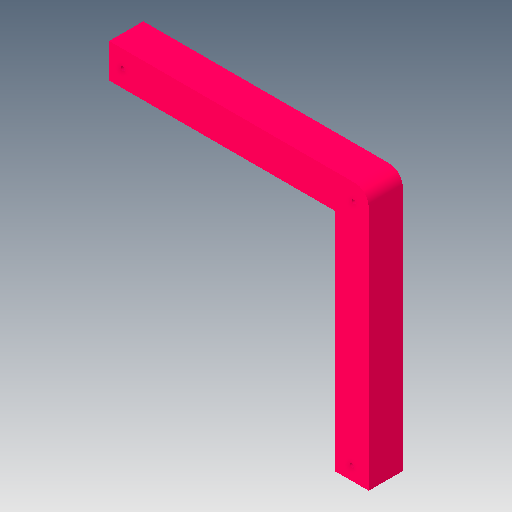
# Autodesk Inventor part: l almini
Saved by Autodesk Inventor 2018 (Build 220112000, 112)
## iProperties
Created: 2019-12-19
Part Number: l almini
Material: Generic
Document SubType Name: Modeling
Designer: Ibnu
Density: 1 g/cm^3
Appearance: Default
Mass: 220.808 g
Surface Area: 372.642 cm^2
Volume: 220.808 cm^3
Author: Ibnu
Autodesk Inventor part; units mm, degrees
ref_plane "YZ Plane" through (0, 0, 0) normal (1, 0, 0) x (0, 1, 0)
ref_plane "XZ Plane" through (0, 0, 0) normal (0, 1, 0) x (-1, 0, 0)
ref_plane "XY Plane" through (0, 0, 0) normal (0, 0, 1) x (1, 0, 0)
sketch "Sketch1" plane through (0, 0, 0) normal (0, 0, 1) x (1, 0, 0)
  line L0 (0, 0) -> (0, 25)
  line L1 (0, 25) -> (165, 25)
  line L2 (165, 0) -> (0, 0)
  line L3 (190, 0) -> (190, -165)
  line L4 (190, -165) -> (165, -165)
  line L5 (165, -165) -> (165, 0)
  line L6 (165, 25) -> (180, 25)
  line L7 (190, 15) -> (190, 0)
  circle A0 centre (10, 12.5) radius 1.5
  circle A1 centre (177.5, -155) radius 1.5
  circle A2 centre (179, 12.5) radius 1.5
  arc A3 (190, 23) -> (188, 25) centre (188, 23) ccw
  arc A4 (190, 15) -> (180, 25) centre (180, 15) ccw
  dimension "d0" = 25
  dimension "d1" = 165
  dimension "d2" = 25
  dimension "d3" = 165
  dimension "d6" = 3
  dimension "d7" = 3
  dimension "d8" = 3
  dimension "d9" = 2
  dimension "d10" = 10
  constraints: 16 end point, 5 centre point, 4 point on circle, 4 tangent, 3 perpendicular, 2 point on line, 1 horizontal, 1 parallel, 1 vertical
  measures "d0" distance of L0.start L0.end
  measures "d1" distance of L0.end L1.end
  measures "d2" distance of L3.end L4.end
  measures "d3" distance of L3.start L3.end
  measures "d6" diameter of A0
  measures "d7" diameter of A1
  measures "d8" diameter of A2
  measures "d9" radius of A3
  measures "d10" radius of A4
extrude "Extrusion1" add sketch "Sketch1" along normal blind 25
body "Solid1"
